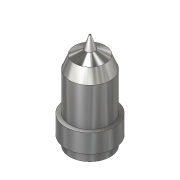
# Autodesk Inventor part: 00_objectivelens_10x
Saved by Autodesk Inventor 2019.4 (Build 234330000, 330)
## iProperties
Created: 2020-11-20
Part Number: 00_objectivelens_10x
Material: Generic
Document SubType Name: Modeling
Designer: diederichbenedict
Density: 1 g/cm^3
Appearance: Chrome - Polished
Author: diederichbenedict
Autodesk Inventor part; units mm, degrees
ref_plane "YZ Plane" through (0, 0, 0) normal (1, 0, 0) x (0, 1, 0)
ref_plane "XZ Plane" through (0, 0, 0) normal (0, 1, 0) x (-1, 0, 0)
ref_plane "XY Plane" through (0, 0, 0) normal (0, 0, 1) x (1, 0, 0)
sketch "Sketch1" plane through (0, 0, 0) normal (0, 0, 1) x (1, 0, 0)
  line L0 (0, -16.2697) -> (0, 26.8303)
  line L1 (0, -16.2697) -> (10.125, -16.2697)
  line L2 (10.125, -16.2697) -> (10.125, -11.5997)
  line L3 (10.125, -11.5997) -> (12.15, -11.5997)
  line L4 (12.15, -11.5997) -> (12.15, -2.3297)
  line L5 (12.15, -2.3297) -> (10.125, -2.3297)
  line L6 (10.125, -2.3297) -> (10.125, 16.8803)
  line L7 (10.125, 16.8803) -> (7.73, 23.0903)
  line L8 (7.73, 23.0903) -> (2.4142, 25.6622)
  line L9 (2.5391, 25.6018) -> (2.4142, 25.6622)
  line L10 (0, 31.6595) -> (0, 26.8303)
  line L11 (0, 31.6595) -> (0.4457, 31.6595)
  line L12 (0.4457, 31.6595) -> (2.4142, 25.6622)
  point P0 (0, 0)
  dimension "d0" = 43.1
  dimension "d1" = 10.125
  dimension "d2" = 4.67
  dimension "d3" = 2.025
  dimension "d4" = 90
  dimension "d5" = 9.27
  dimension "d6" = 19.21
  dimension "d7" = 7.73
  dimension "d8" = 39.36
  constraints: 26 end point, 4 perpendicular, 2 horizontal, 2 point on line, 2 vertical, 1 collinear
  measures "d0" distance of L0.start L0.end
  measures "d1" distance of L0.start L1.end
  measures "d2" distance of L1.end L2.end
  measures "d3" distance of L2.end L3.end
  measures "d4" angle of L2 L3
  measures "d5" distance of L3.end L4.end
  measures "d6" distance of L5.end L6.end
  measures "d7" distance from line of L0 L7.end
  measures "d8" distance from line of L1 L7.end
revolve "Revolution1" add sketch "Sketch1" angle 360 about axis through (0, -16.2697, 0) along (0, 1, 0)
body "Solid1"
